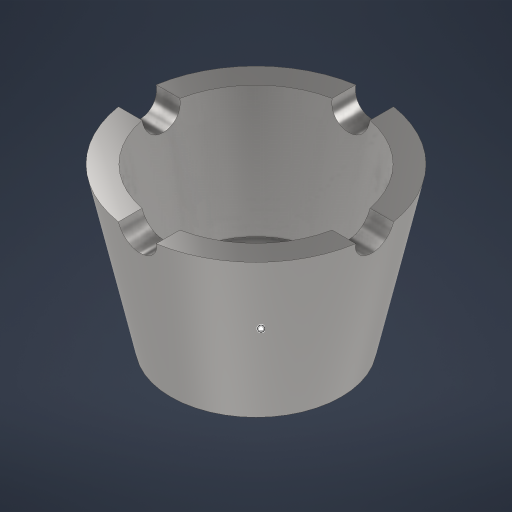
# Autodesk Inventor part: cup
Saved by Autodesk Inventor 2023 (Build 270158000, 158)
## iProperties
Created: 2023-03-09
Part Number: cup
Material: Steel, Cast
Document SubType Name: Modeling
Designer: kamraj
Density: 7.85 g/cm^3
Appearance: Semi-Polished
Author: kamraj
Autodesk Inventor part; units mm, degrees
ref_plane "YZ Plane" through (0, 0, 0) normal (1, 0, 0) x (0, 1, 0)
ref_plane "XZ Plane" through (0, 0, 0) normal (0, 1, 0) x (-1, 0, 0)
ref_plane "XY Plane" through (0, 0, 0) normal (0, 0, 1) x (1, 0, 0)
sketch "Sketch3" plane through (0, 0, 0) normal (0, 0, 1) x (1, 0, 0)
  line L0 (0, 0) -> (0, 42)
  line L1 (11.25, 0) -> (11.25, 12)
  line L2 (11.25, 12) -> (19, 12)
  line L3 (19, 12) -> (25.6098, 42)
  line L4 (25.6098, 42) -> (31.7537, 42)
  line L5 (31.7537, 42) -> (22.5, 0)
  line L6 (22.5, 0) -> (11.25, 0)
  dimension "d3" = 6
  dimension "d4" = 42
  dimension "d5" = 12
  dimension "d6" = 22.5
  dimension "d7" = 45
  dimension "d8" = 38
  dimension "d9" = 63.5073
  constraints: 14 end point, 3 parallel, 2 vertical, 1 perpendicular, 1 point on line
  measures "d3" distance between parallel lines of L5 L3
  measures "d4" distance between parallel lines of L6 L4
  measures "d5" distance between parallel lines of L6 L2
  measures "d6" diameter of L1 L0
  measures "d7" diameter of L5.end L0
  measures "d8" diameter of L2.end L0
  measures "d9" diameter of L4.end L0
revolve "Revolution1" add sketch "Sketch3" angle 360 about axis through (0, 0, 0) along (0, 1, 0)
sketch "Sketch4" plane through (0, 0, 0) normal (0, 0, 1) x (1, 0, 0)
  line L0 (31.7537, 42) -> (-31.7537, 42) projected
  circle A0 centre (0, 42) radius 5
  point P0 (0, 0)
  dimension "d11" = 10
  constraints: 1 centre point, 1 midpoint
  measures "d11" diameter of A0
extrude "Extrusion2" cut sketch "Sketch4" along normal through all
pattern_circular "Circular Pattern1" count 4 over 360 about axis through (0, -10, 0) along (0, 1, 0) of "Extrusion2"
